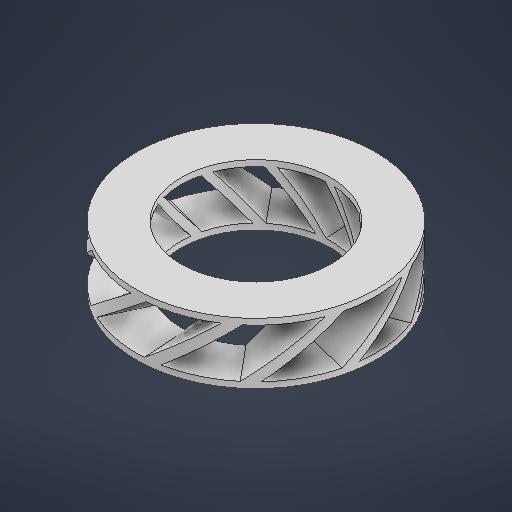
# Autodesk Inventor part: spring
Saved by Autodesk Inventor 2025.2 (Build 292293000, 293)
## iProperties
Created: 2025-05-23
Part Number: spring
Material: Generic
Document SubType Name: Modeling
Designer: klawy
Density: 1 g/cm^3
Appearance: Default
Author: klawy
Autodesk Inventor part; units mm, degrees
ref_plane "YZ Plane" through (0, 0, 0) normal (1, 0, 0) x (0, 1, 0)
ref_plane "XZ Plane" through (0, 0, 0) normal (0, 1, 0) x (-1, 0, 0)
sketch "Sketch1" plane through (0, 0, 0) normal (0, 1, 0) x (-1, 0, 0)
  circle A0 centre (0, 0) radius 12.55
  circle A1 centre (0, 0) radius 20
  dimension "d0" = 25.1
  dimension "d1" = 40
  constraints: 2 centre point, 2 coincident
  measures "d0" diameter of A0
  measures "d1" diameter of A1
extrude "Extrusion1" add sketch "Sketch1" along normal blind 1
ref_plane "Work Plane3" through (0, 5.1, 0) normal (0, -1, 0) x (1, 0, 0)
ref_plane "Work Plane1" through (0, 10.2, 0) normal (0, 1, 0) x (1, 0, 0)
ref_plane "Work Plane2" through (0, 0, 0) normal (0, -1, 0) x (1, 0, 0)
mirror "Mirror1" about plane through (0, 5.1, 0) normal (0, -1, 0) of "Extrusion1"
sketch "Sketch3" plane through (0, 0, 0) normal (1, 0, 0) x (0, 1, 0)
  line L0 (0, -20) -> (0, 20) projected
  line L1 (0, 20) -> (-2, 20)
  line L2 (-2, 20) -> (-2, 12.55)
  line L3 (-2, 12.55) -> (0, 12.55)
  line L4 (0, 12.55) -> (0, 20)
  line L5 (1, 12.55) -> (1, -12.55) projected
  line L6 (0, 12.55) -> (0, -12.55) projected
  point P0 (0, 0)
  dimension "d6" = 2
  constraints: 8 end point, 2 parallel, 1 horizontal, 1 perpendicular, 1 point on line
  measures "d6" distance between parallel lines of L0 L2
coil "Coil1" sketch "Sketch3" operation add axis through (0, -10, 0) along (0, 1, 0) pitch 100 turns 0.2 hand right
pattern_circular "Circular Pattern1" count 10 over 360 about axis through (0, -10, 0) along (0, 1, 0) of "Coil1"
split "Split1" plane through (0, 10.2, 0) removes the side toward (0, 1, 0)
split "Split2" plane through (0, 0, 0) removes the side toward (0, -1, 0)
body "Solid1"
